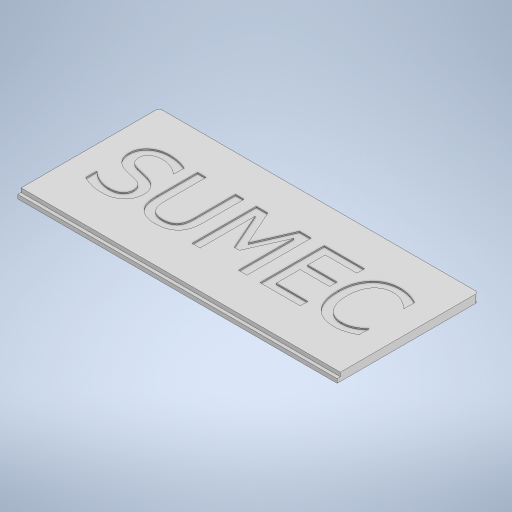
# Autodesk Inventor part: Kryt těla
Saved by Autodesk Inventor 2023.2 (Build 272271030, 271C)
## iProperties
Created: 2023-03-18
Part Number: Kryt těla
Material: Všeobecné
Document SubType Name: Modeling
Designer: jaryj
Density: 1 g/cm^3
Appearance: Výchozí
Author: jaryj
Autodesk Inventor part; units mm, degrees
ref_plane "YZ Plane" through (0, 0, 0) normal (1, 0, 0) x (0, 1, 0)
ref_plane "XZ Plane" through (0, 0, 0) normal (0, 1, 0) x (-1, 0, 0)
ref_plane "XY Plane" through (0, 0, 0) normal (0, 0, 1) x (1, 0, 0)
sketch "Náčrt1" plane through (0, 0, 0) normal (0, 1, 0) x (-1, 0, 0)
  line L0 (0, 0) -> (49.75, 0)
  line L1 (49.75, 0) -> (49.75, -44)
  line L2 (49.75, -44) -> (0, -44)
  line L3 (0, -44) -> (0, 0)
  line L4 (0, -1) -> (49.75, -1)
  line L5 (18, -41) -> (16, -41)
  line L6 (18, -41) -> (18, -43.9)
  line L7 (18, -43.9) -> (16, -43.9)
  line L8 (16, -43.9) -> (16, -41)
  line L9 (5.25, -44) -> (5.25, -40)
  line L10 (5.25, -40) -> (9.75, -40)
  line L11 (9.75, -40) -> (9.75, -44)
  dimension "d0" = 44
  dimension "d1" = 49.75
  dimension "d2" = 1
  dimension "d5" = 3
  dimension "d16" = 0.1
  dimension "d17" = 31.75
  dimension "d18" = 2
  dimension "d28" = 4.5
  dimension "d29" = 4
  dimension "d30" = 5.25
  constraints: 24 end point, 7 perpendicular, 4 point on line, 2 parallel, 1 horizontal, 1 vertical
  measures "d0" distance of L2.end L0.start
  measures "d1" distance of L1.end L2.end
  measures "d2" distance between parallel lines of L0 L4
  measures "d5" distance between parallel lines of L2 L5
  measures "d16" distance between parallel lines of L2 L7
  measures "d17" distance from line of L1 L5.start
  measures "d18" distance of L5.start L5.end
  measures "d28" distance of L9.end L10.end
  measures "d29" distance of L10.end L11.end
  measures "d30" distance between parallel lines of L3 L9
extrude "Vysunutí1" add sketch "Náčrt1" along normal blind 2.5 contours L4 L1 L2 L11 L10 L9 L3 | L9 L10 L11 L2 | L6 L7 L8 L5
extrude "Vysunutí2" add sketch "Náčrt1" along normal blind 1.25 contours L0 L1 L4 L3
extrude "Vysunutí3" add sketch "Náčrt1" against normal blind 7.5 contours L6 L7 L8 L5
sketch "Náčrt3" plane through (-16, 0, -43.9) normal (0, 0, -1) x (-1, 0, 0)
  line L0 (0, 0) -> (0, -7.5) projected
  line L1 (2, -7.5) -> (0, -7.5) projected
  line L2 (2, 0) -> (2, -7.5) projected
  line L3 (0, 0) -> (0, -7.5) projected
  line L4 (0, -5.6) -> (2, -5.6)
  line L5 (2, 0) -> (2, -7.5) projected
  point P0 (-16, 0)
  dimension "d19" = 1.9
  constraints: 2 end point, 2 point on line, 1 perpendicular
  measures "d19" distance between parallel lines of L4 L1
extrude "Vysunutí5" add sketch "Náčrt3" along normal blind 5
fillet "Zaoblení1" radius 1 1 edges at (-49.75, 1.25, -44)
extrude "Vysunutí6" add sketch "Náčrt1" against normal blind 8 contours L9 L10 L11 L2
sketch "Náčrt7" plane through (-5.25, -8, -40) normal (1, 0, 0) x (0, 0, -1)
  line L0 (0, 8) -> (0, 0) projected
  line L1 (4, 0) -> (0, 0) projected
  line L2 (4, 8) -> (4, 0) projected
  line L3 (0, 8) -> (0, 0) projected
  line L4 (0, 2) -> (4, 2)
  line L5 (4, 8) -> (4, 0) projected
  point P0 (-40, 8)
  dimension "d36" = 2
  constraints: 2 end point, 2 point on line, 1 perpendicular
  measures "d36" distance between parallel lines of L1 L4
extrude "Vysunutí8" add sketch "Náčrt7" along normal up to surface (5.25 mm away)
sketch "Náčrt8" plane through (0, 0, -44) normal (0, 0, -1) x (-1, 0, 0)
  line L0 (9.75, 0) -> (9.75, -8) projected
  line L1 (5.25, -6) -> (0, -6) projected
  point P0 (0, 0)
  point P1 (7.5, -3)
  dimension "d46" = 2.25
  dimension "d47" = 3
  measures "d46" distance from line of L0 point (7.5, -3)
  measures "d47" distance from line of L1 point (7.5, -3)
hole "Díra1" at (-7.5, -3, -44) direction (0, 0, 1) diameter 2 end through all
mirror "Zrcadlit2" about plane through (0, 0, -1) normal (1, 0, 0)
sketch "Náčrt4" plane through (0, 2.5, 0) normal (0, 1, 0) x (1, 0, 0)
  line L0 (-43.5, 33) -> (41.5, 33) construction
  line L1 (41.5, 33) -> (41.5, 13) construction
  line L2 (41.5, 13) -> (-43.5, 13) construction
  line L3 (-43.5, 13) -> (-43.5, 33) construction
  line L4 (-48.75, 44) -> (48.75, 44) projected
  line L5 (-49.75, 43) -> (-49.75, 1) projected
  spline S0 degree 2 poles (-35.8987, 12.2869) (-38.0705, 12.2869) (-41.1175, 13.1945) (-42.4627, 13.8428) knots 0 0 0 1 2 2 2
  line L6 (-42.4627, 13.8428) -> (-42.4627, 17.1815)
  line L7 (-42.4627, 17.1815) -> (-42.2682, 17.1815)
  spline S1 degree 2 poles (-42.2682, 17.1815) (-40.9554, 15.9498) (-37.6329, 14.5883) (-36.0932, 14.5883) knots 0 0 0 1 2 2 2
  spline S2 degree 2 poles (-36.0932, 14.5883) (-33.889, 14.5883) (-31.6361, 16.4198) (-31.6361, 17.9271) knots 0 0 0 1 2 2 2
  spline S3 degree 2 poles (-31.6361, 17.9271) (-31.6361, 19.1264) (-32.8193, 20.6175) (-34.0997, 20.9903) knots 0 0 0 1 2 2 2
  spline S4 degree 2 poles (-34.0997, 20.9903) (-35.0235, 21.2496) (-36.5632, 21.6062) (-37.7139, 21.8979) knots 0 0 0 1 2 2 2
  spline S5 degree 2 poles (-37.7139, 21.8979) (-38.7512, 22.1734) (-40.3882, 23) (-41.0203, 23.6645) knots 0 0 0 1 2 2 2
  spline S6 degree 2 poles (-41.0203, 23.6645) (-41.6361, 24.329) (-42.3169, 26.1118) (-42.3169, 27.2788) knots 0 0 0 1 2 2 2
  spline S7 degree 2 poles (-42.3169, 27.2788) (-42.3169, 29.7099) (-38.5243, 33) (-35.5908, 33) knots 0 0 0 1 2 2 2
  spline S8 degree 2 poles (-35.5908, 33) (-33.9052, 33) (-30.923, 32.3355) (-29.6426, 31.7034) knots 0 0 0 1 2 2 2
  line L8 (-29.6426, 31.7034) -> (-29.6426, 28.5267)
  line L9 (-29.6426, 28.5267) -> (-29.8371, 28.5267)
  spline S9 degree 2 poles (-29.8371, 28.5267) (-30.7934, 29.4019) (-33.7755, 30.6985) (-35.4125, 30.6985) knots 0 0 0 1 2 2 2
  spline S10 degree 2 poles (-35.4125, 30.6985) (-37.2601, 30.6985) (-39.5454, 28.9643) (-39.5454, 27.5543) knots 0 0 0 1 2 2 2
  spline S11 degree 2 poles (-39.5454, 27.5543) (-39.5454, 26.2901) (-38.2002, 24.7828) (-36.936, 24.4425) knots 0 0 0 1 2 2 2
  spline S12 degree 2 poles (-36.936, 24.4425) (-36.0932, 24.2156) (-33.6459, 23.6321) (-32.8355, 23.389) knots 0 0 0 1 2 2 2
  spline S13 degree 2 poles (-32.8355, 23.389) (-30.7771, 22.7569) (-28.8647, 20.2123) (-28.8647, 18.3485) knots 0 0 0 1 2 2 2
  spline S14 degree 2 poles (-28.8647, 18.3485) (-28.8647, 17.1653) (-29.8209, 14.8963) (-30.6799, 14.1021) knots 0 0 0 1 2 2 2
  spline S15 degree 2 poles (-30.6799, 14.1021) (-31.6361, 13.2269) (-34.0673, 12.2869) (-35.8987, 12.2869) knots 0 0 0 1 2 2 2
  spline S16 degree 2 poles (-19.1726, 12.222) (-20.9392, 12.222) (-23.5648, 13.1459) (-24.4887, 14.0697) knots 0 0 0 1 2 2 2
  spline S17 degree 2 poles (-24.4887, 14.0697) (-25.5421, 15.107) (-26.4011, 18.0243) (-26.4011, 20.1637) knots 0 0 0 1 2 2 2
  line L10 (-26.4011, 20.1637) -> (-26.4011, 32.6434)
  line L11 (-26.4011, 32.6434) -> (-23.7431, 32.6434)
  line L12 (-23.7431, 32.6434) -> (-23.7431, 20.1637)
  spline S18 degree 2 poles (-23.7431, 20.1637) (-23.7431, 18.7699) (-23.3865, 16.8898) (-22.8841, 16.128) knots 0 0 0 1 2 2 2
  spline S19 degree 2 poles (-22.8841, 16.128) (-22.3493, 15.3177) (-20.5016, 14.4911) (-19.1726, 14.4911) knots 0 0 0 1 2 2 2
  spline S20 degree 2 poles (-19.1726, 14.4911) (-17.9246, 14.4911) (-15.9797, 15.3177) (-15.4449, 16.128) knots 0 0 0 1 2 2 2
  spline S21 degree 2 poles (-15.4449, 16.128) (-14.9425, 16.8898) (-14.5859, 18.7536) (-14.5859, 20.0989) knots 0 0 0 1 2 2 2
  line L13 (-14.5859, 20.0989) -> (-14.5859, 32.6434)
  line L14 (-14.5859, 32.6434) -> (-11.9279, 32.6434)
  line L15 (-11.9279, 32.6434) -> (-11.9279, 20.1637)
  spline S22 degree 2 poles (-11.9279, 20.1637) (-11.9279, 18.0729) (-12.7707, 15.0908) (-13.8404, 14.0697) knots 0 0 0 1 2 2 2
  spline S23 degree 2 poles (-13.8404, 14.0697) (-14.7966, 13.1297) (-17.325, 12.222) (-19.1726, 12.222) knots 0 0 0 1 2 2 2
  line L16 (9.0284, 12.6434) -> (6.3703, 12.6434)
  line L17 (6.3703, 12.6434) -> (6.3703, 29.872)
  line L18 (6.3703, 29.872) -> (1.1515, 18.154)
  line L19 (1.1515, 18.154) -> (-0.4692, 18.154)
  line L20 (-0.4692, 18.154) -> (-5.6394, 29.872)
  line L21 (-5.6394, 29.872) -> (-5.6394, 12.6434)
  line L22 (-5.6394, 12.6434) -> (-8.1191, 12.6434)
  line L23 (-8.1191, 12.6434) -> (-8.1191, 32.6434)
  line L24 (-8.1191, 32.6434) -> (-4.4887, 32.6434)
  line L25 (-4.4887, 32.6434) -> (0.5032, 21.5089)
  line L26 (0.5032, 21.5089) -> (5.3331, 32.6434)
  line L27 (5.3331, 32.6434) -> (9.0284, 32.6434)
  line L28 (9.0284, 32.6434) -> (9.0284, 12.6434)
  line L29 (13.0802, 12.6434) -> (13.0802, 32.6434)
  line L30 (13.0802, 32.6434) -> (25.5924, 32.6434)
  line L31 (25.5924, 32.6434) -> (25.5924, 30.2771)
  line L32 (25.5924, 30.2771) -> (15.7382, 30.2771)
  line L33 (15.7382, 30.2771) -> (15.7382, 24.799)
  line L34 (15.7382, 24.799) -> (24.9279, 24.799)
  line L35 (24.9279, 24.799) -> (24.9279, 22.4327)
  line L36 (24.9279, 22.4327) -> (15.7382, 22.4327)
  line L37 (15.7382, 22.4327) -> (15.7382, 15.0097)
  line L38 (15.7382, 15.0097) -> (25.5924, 15.0097)
  line L39 (25.5924, 15.0097) -> (25.5924, 12.6434)
  line L40 (25.5924, 12.6434) -> (13.0802, 12.6434)
  spline S24 degree 2 poles (36.3217, 12.2869) (34.3768, 12.2869) (31.0867, 13.5997) (29.8874, 14.9125) knots 0 0 0 1 2 2 2
  spline S25 degree 2 poles (29.8874, 14.9125) (28.688, 16.2091) (27.3752, 20.0989) (27.3752, 22.6272) knots 0 0 0 1 2 2 2
  spline S26 degree 2 poles (27.3752, 22.6272) (27.3752, 25.1394) (28.6556, 28.8671) (29.8712, 30.2447) knots 0 0 0 1 2 2 2
  spline S27 degree 2 poles (29.8712, 30.2447) (31.0705, 31.59) (34.3444, 33) (36.3703, 33) knots 0 0 0 1 2 2 2
  spline S28 degree 2 poles (36.3703, 33) (37.3752, 33) (39.1418, 32.7083) (39.8874, 32.4814) knots 0 0 0 1 2 2 2
  spline S29 degree 2 poles (39.8874, 32.4814) (40.5357, 32.2707) (41.8809, 31.671) (42.5454, 31.3144) knots 0 0 0 1 2 2 2
  line L41 (42.5454, 31.3144) -> (42.5454, 28.1053)
  line L42 (42.5454, 28.1053) -> (42.3347, 28.1053)
  spline S30 degree 2 poles (42.3347, 28.1053) (41.9781, 28.4295) (40.876, 29.3371) (40.0818, 29.7747) knots 0 0 0 1 2 2 2
  spline S31 degree 2 poles (40.0818, 29.7747) (39.3201, 30.1961) (37.5211, 30.731) (36.3541, 30.731) knots 0 0 0 1 2 2 2
  spline S32 degree 2 poles (36.3541, 30.731) (35.0737, 30.731) (32.7885, 29.6775) (31.9295, 28.6726) knots 0 0 0 1 2 2 2
  spline S33 degree 2 poles (31.9295, 28.6726) (31.0867, 27.6515) (30.1467, 24.5559) (30.1467, 22.6272) knots 0 0 0 1 2 2 2
  spline S34 degree 2 poles (30.1467, 22.6272) (30.1467, 20.5689) (31.1353, 17.6029) (31.9943, 16.5818) knots 0 0 0 1 2 2 2
  spline S35 degree 2 poles (31.9943, 16.5818) (32.8371, 15.5932) (35.09, 14.5883) (36.3541, 14.5883) knots 0 0 0 1 2 2 2
  spline S36 degree 2 poles (36.3541, 14.5883) (37.5049, 14.5883) (39.466, 15.1556) (40.2277, 15.577) knots 0 0 0 1 2 2 2
  spline S37 degree 2 poles (40.2277, 15.577) (40.9571, 15.9984) (42.0429, 16.8736) (42.3509, 17.1815) knots 0 0 0 1 2 2 2
  line L43 (42.3509, 17.1815) -> (42.5454, 17.1815)
  line L44 (42.5454, 17.1815) -> (42.5454, 14.0049)
  spline S38 degree 2 poles (42.5454, 14.0049) (41.8809, 13.6969) (40.7139, 13.1297) (39.8874, 12.8703) knots 0 0 0 1 2 2 2
  spline S39 degree 2 poles (39.8874, 12.8703) (39.0122, 12.5786) (37.5211, 12.2869) (36.3217, 12.2869) knots 0 0 0 1 2 2 2
  point P0 (0, 0)
  dimension "d22" = 85
  dimension "d23" = 20
  dimension "d24" = 11
  dimension "d25" = 6.25
  constraints: 2 other
  measures "d22" distance of L1.end L2.end
  measures "d23" distance of L0.end L1.end
  measures "d24" distance between parallel lines of L4 L0
  measures "d25" distance between parallel lines of L5 L3
emboss "Reliéf1" sketch "Náčrt4" operation cut depth 0.4 direction (0, -1, 0)
